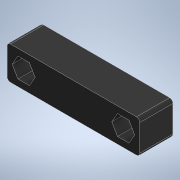
# Autodesk Inventor part: AntennaHolder2
Saved by Autodesk Inventor 2021 (Build 250183000, 183)
## iProperties
Created: 2020-09-13
Part Number: AntennaHolder2
Material: Generic
Document SubType Name: Modeling
Designer: Viktor
Density: 1 g/cm^3
Appearance: Default
Author: Viktor
## iProperties of the stored document _3DPrint.ipt
Created: 2020-10-11
Part Number: _3DPrint
Material: Generic
Document SubType Name: Modeling
Designer: Viktor
Density: 1 g/cm^3
Appearance: Default
Author: Viktor
Autodesk Inventor part; units mm, degrees
note: some values were not read from the file. Chosen so that the rebuilt part matches the saved one: arc direction of "Extrusion2".
ref_plane "YZ Plane" through (0, 0, 0) normal (1, 0, 0) x (0, 1, 0)
ref_plane "XZ Plane" through (0, 0, 0) normal (0, 1, 0) x (-1, 0, 0)
sketch "Sketch1" plane through (0, 0, 0) normal (0, 0, 1) x (1, 0, 0)
  line L0 (-20, -5) -> (20, -5)
  line L1 (20, -5) -> (20, 5)
  line L2 (20, 5) -> (-20, 5)
  line L3 (-20, 5) -> (-20, -5)
  line L4 (-20, -5) -> (20, 5) construction
  line L5 (20, -5) -> (-20, 5) construction
  point P0 (0, 0)
  dimension "d0" = 10
  dimension "d1" = 40
  constraints: 12 end point, 2 midpoint, 2 parallel, 1 horizontal, 1 perpendicular
  measures "d0" distance of L2.end L0.start
  measures "d1" distance of L1.end L2.end
extrude "Extrusion1" add sketch "Sketch1" along normal blind 10
sketch "Sketch2" plane through (0, 0, 10) normal (0, 0, 1) x (1, 0, 0)
  line L0 (-28, 0) -> (28, 0) projected
  circle A0 centre (-15, 0) radius 1.85
  circle A1 centre (15, 0) radius 1.85
  point P0 (0, 0)
  point P1 (16.85, 0)
  point P2 (13.15, 0)
  dimension "d4" = 3.7
  dimension "d5" = 3.7
  dimension "d6" = 15
  dimension "d7" = 15
  constraints: 2 centre point, 2 point on line
  measures "d4" diameter of A0
  measures "d5" diameter of A1
  measures "d6" distance of point (0, 0) A0.centre
  measures "d7" distance of point (0, 0) A1.centre
extrude "Extrusion2" cut sketch "Sketch2" against normal through all
chamfer "Chamfer1" distance 9 angle 45 1 edges at (0, -5, 10)
ref_plane "Work Plane1" through (0, 0, 2) normal (0, 0, -1) x (-1, 0, 0)
sketch "Sketch3" plane through (0, 0, 2) normal (0, 0, -1) x (-1, 0, 0)
  circle A0 centre (15, 0) radius 1.85 projected
  circle A1 centre (-15, 0) radius 1.85 projected
  line L0 (11.5359, 0) -> (13.2679, 3)
  line L1 (13.2679, 3) -> (16.7321, 3)
  line L2 (16.7321, 3) -> (18.4641, 0)
  line L3 (18.4641, 0) -> (16.7321, -3)
  line L4 (16.7321, -3) -> (13.2679, -3)
  line L5 (13.2679, -3) -> (11.5359, 0)
  line L6 (-18.4641, 0) -> (-16.7321, 3)
  line L7 (-16.7321, 3) -> (-13.2679, 3)
  line L8 (-13.2679, 3) -> (-11.5359, 0)
  line L9 (-11.5359, 0) -> (-13.2679, -3)
  line L10 (-13.2679, -3) -> (-16.7321, -3)
  line L11 (-16.7321, -3) -> (-18.4641, 0)
  point P0 (0, 0)
  point P1 (15, 3)
  dimension "d14" = 6
  dimension "d15" = 6
  constraints: 24 end point, 2 coincident, 2 horizontal, 1 midpoint, 26 other
  measures "d14" distance between parallel lines of L4 L1
  measures "d15" distance between parallel lines of L10 L7
extrude "Extrusion3" cut sketch "Sketch3" against normal up to surface contours A1 | L0 L1 L2 L3 L4 L5 | L6 L7 L8 L9 L10 L11 surface through (-10, -0.5, 5.5) normal (0, -0.7071068, 0.7071068)
fillet "Fillet1" radius 1 4 edges at (20, 5, 5) (20, -5, 0.5) (-20, 5, 5) (-20, -5, 0.5)
sketch "Sketch4" plane through (0, 0, 10) normal (0, 0, 1) x (1, 0, 0)
  line L0 (16.7321, 3) -> (18.4641, 0) projected
  line L1 (18.4641, 0) -> (16.7321, -3) projected
  line L2 (16.7321, -3) -> (13.2679, -3) projected
  line L3 (13.2679, -3) -> (11.5359, 0) projected
  line L4 (11.5359, 0) -> (13.2679, 3) projected
  line L5 (13.2679, 3) -> (16.7321, 3) projected
  line L6 (-16.7321, 3) -> (-13.2679, 3) projected
  line L7 (-13.2679, 3) -> (-11.5359, 0) projected
  line L8 (-11.5359, 0) -> (-13.2679, -3) projected
  line L9 (-13.2679, -3) -> (-16.7321, -3) projected
  line L10 (-16.7321, -3) -> (-18.4641, 0) projected
  line L11 (-18.4641, 0) -> (-16.7321, 3) projected
  arc A0 (-20, -4) -> (-19, -5) centre (-19, -4) ccw projected
  line L12 (-19, -5) -> (19, -5) projected
  arc A1 (19, -5) -> (20, -4) centre (19, -4) ccw projected
  line L13 (20, -4) -> (20, 4) projected
  line L14 (20, 4) -> (-20, 4) projected
  line L15 (-20, 4) -> (-20, -4) projected
  point P0 (0, 0)
extrude "Extrusion4" add sketch "Sketch4" against normal up to surface surface through (-10, -0.5, 5.5) normal (0, -0.7071068, 0.7071068)
equation "\"d5\" = d4"
equation "\"d7\" = d6"
equation "\"d15\" = d14"
body "Solid1"
